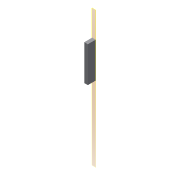
# Autodesk Inventor part: EjectionRamp
Saved by Autodesk Inventor 2018 (Build 220112000, 112)
## iProperties
Created: 2018-12-23
Part Number: EjectionRamp
Material: Generic
Document SubType Name: Modeling
Designer: ball
Density: 1 g/cm^3
Appearance: Default
Author: ball
Autodesk Inventor part; units mm, degrees
ref_plane "YZ Plane" through (0, 0, 0) normal (1, 0, 0) x (0, 1, 0)
ref_plane "XZ Plane" through (0, 0, 0) normal (0, 1, 0) x (-1, 0, 0)
ref_plane "XY Plane" through (0, 0, 0) normal (0, 0, 1) x (1, 0, 0)
ref_plane "Work Plane1" through (0, 0, 0) normal (0, 0, 1) x (1, 0, 0)
sketch "Sketch1" plane through (0, 0, 0) normal (0, 0, 1) x (1, 0, 0)
  line L0 (16, 228) -> (4, 228) construction
  line L1 (4, 148) -> (-8, 148) construction
  line L2 (4, 228) -> (-4.0164, 228)
  line L3 (-4.0164, 228) -> (-4.0164, 148)
  line L4 (-4.0164, 148) -> (4, 148)
  line L5 (4, 148) -> (4, 228)
  point P0 (0, 0)
  constraints: 12 end point, 3 horizontal, 2 parallel, 1 perpendicular, 1 point on line, 4 other
extrude "Extrusion1" add sketch "Sketch1" along normal blind 17.78
sketch "Sketch2" plane through (-4.0164, 148, 0) normal (0, -1, 0) x (1, 0, 0)
  line L0 (0, 17.78) -> (8.0164, 17.78) construction
  line L1 (0, 0) -> (0, 17.78) construction
  line L2 (0, 0) -> (0, 17.78) projected
  line L3 (8.0164, 17.78) -> (0, 17.78) projected
  line L4 (0, 0) -> (0, 17.78)
  line L5 (0, 17.78) -> (5.969, 17.78)
  line L6 (5.969, 17.78) -> (0, 0)
  point P0 (4.0164, 0)
  dimension "d2" = 5.969
  constraints: 6 end point, 1 perpendicular, 1 point on line
  measures "d2" distance of L0.start L5.end
extrude "Extrusion2" cut sketch "Sketch2" against normal up to surface (80 mm away)
sketch "Sketch3" plane through (0, 0, 0) normal (0, 0, -1) x (-1, 0, 0)
  circle A0 centre (0, 220) radius 2 construction
  circle A1 centre (0, 156) radius 2 construction
  circle A2 centre (0, 188) radius 2 construction
  point P0 (0, 0)
  constraints: 3 centre point, 6 other
hole "Hole1" at (0, 220, 0) at (0, 188, 0) at (0, 156, 0) direction (0, 0, 1) diameter 3.937 depth 6.35
body "Solid1"
